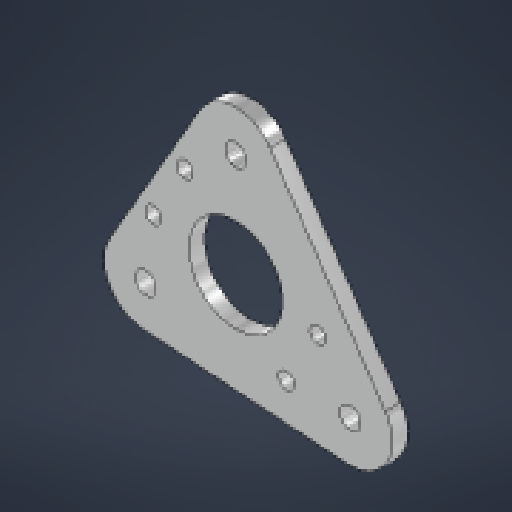
# Autodesk Inventor part: PLATE,TURRET,MOTOR,MOUNT
Saved by Autodesk Inventor 2026.1 (Build 301233020, 233B)
## iProperties
Created: 2026-02-09
Part Number: PLATE,TURRET,MOTOR,MOUNT
Material: Aluminum 6061
Document SubType Name: Sheet Metal
Designer: littl
Density: 2.7 g/cm^3
Sheet Metal Rule: Default
Appearance: Aluminum - Flat
Author: littl
Autodesk Inventor part; units mm, degrees
ref_plane "YZ Plane" through (0, 0, 0) normal (1, 0, 0) x (0, 1, 0)
ref_plane "XZ Plane" through (0, 0, 0) normal (0, 1, 0) x (-1, 0, 0)
ref_plane "XY Plane" through (0, 0, 0) normal (0, 0, 1) x (1, 0, 0)
sketch "Sketch2" plane through (0, 0, 0) normal (0, 0, 1) x (1, 0, 0)
  line L0 (27.4963, -15.875) -> (0, 0) construction
  arc A0 (-38.4948, -9.525) -> (-28.3934, -28.5433) centre (-27.4963, -15.875) ccw
  arc A1 (10.5225, 38.861) -> (-10.9985, 38.1) centre (0, 31.75) ccw
  line L1 (-38.4948, -9.525) -> (-10.9985, 38.1)
  line L2 (10.5225, 38.861) -> (45.7067, -13.2026)
  line L3 (34.2871, -32.9819) -> (-28.3934, -28.5433)
  circle A2 centre (-182.5755, 105.41) radius 190.5 construction
  line L4 (-182.5755, 105.41) -> (0, 0) construction
  line L5 (-133.2704, -78.5989) -> (50.7384, -29.2938) construction
  line L6 (50.7384, -29.2938) -> (1.4334, 154.715) construction
  line L7 (50.7384, -29.2938) -> (0, 0) construction
  arc A3 (34.2871, -32.9819) -> (45.7067, -13.2026) centre (35.1842, -20.3136) ccw
  point P0 (0, 0)
  point P1 (-25.1827, 3.3154)
  point P2 (-20.1512, -15.4625)
  point P3 (-3.3154, -25.1827)
  point P4 (15.4625, -20.1512)
  point P5 (25.1827, -3.3154)
  point P6 (20.1512, 15.4625)
  point P7 (3.3154, 25.1827)
  point P8 (-15.4625, 20.1512)
  dimension "d74" = 31.75
  dimension "d77" = 360
  dimension "d80" = 25.4
  dimension "d83" = 360
  dimension "d96" = 381
  dimension "d97" = 210.82
  dimension "d98" = 12.7
  dimension "d99" = 12.7
  dimension "d100" = 12.7
  constraints: 16 end point, 8 point on circle, 8 tangent, 4 centre point, 4 coincident, 2 equal radius, 2 symmetric about line, 1 collinear, 1 perpendicular, 1 vertical alignment, 13 other
  measures "d74" distance of point (0, 0) point (0, 31.75)
  measures "d80" distance of point (0, 0) point (-25.183, 3.315)
  measures "d96" diameter of A2
  measures "d97" distance of L4.start L0.end
  measures "d98" distance from line of L5 point (35.184, -20.314)
  measures "d99" distance from line of L6 point (35.184, -20.314)
  measures "d100" radius of A3
extrude "Plate2" add sketch "Sketch2" along normal blind 4.7625
hole "Hole3" at (35.1842, -20.3136, 0) at (-27.4963, -15.875, 0) at (0, 31.75, 0) direction (0, 0, 1) diameter 6.5278 end through all clearance for "Flat Head Machine Screw (82)" size "1/4" standard "Ansi Unified Screw Threads"
hole "Hole4" at (0, 0, 0) direction (0, 0, 1) diameter 28.575 end through all
hole "Hole5" at (-25.1827, 3.3154, 0) at (15.4625, -20.1512, 0) at (25.1827, -3.3154, 0) at (-15.4625, 20.1512, 0) direction (0, 0, 1) diameter 4.9784 end through all clearance for "Flat Head Machine Screw (82)" size "#10" standard "Ansi Unified Screw Threads"
equation "\"BendRadius\" = Thickness"
equation "\"BendReliefWidth\" = Thickness"
equation "\"BendReliefDepth\" = 0.5 * Thickness"
equation "\"CornerReliefSize\" = 4 * Thickness"
equation "\"MinimumRemnant\" = 2 * Thickness"
equation "\"TransitionRadius\" = BendRadius"
equation "\"JacobiRadiusSize\" = BendRadius"
equation "\"GapSize\" = Thickness"
equation "\"Thickness\" = 4.7625"
body "Solid2"
